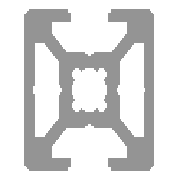
# Autodesk Inventor part: 3 842 993 422-25mm
Saved by Autodesk Inventor 2011 SP1 (Build 150282100, 282)
## iProperties
Created: 2011-02-10
Part Number: 3 842 993 422-25mm
Document SubType Name: Modeling
Designer: S. Wile
Density: 2.71 g/cm^3
Categories: <MemberInstance><Categories><Category DisplayName="Structural Shapes" InternalName="089c4875-fa83-4c05-b084-43b9cc11f5ed" Mnemonic="GRDR"><CategoryParameter DisplayName="Custom Base Point" InternalName="4f1d1b73-316d-484b-a3df-9cbabb16eb77" Mnemonic="shpBasePoint"/><CategoryParameter DisplayName="FG Authored" InternalName="9c666724-f362-4ea7-ac62-f6a007de5c69" Mnemonic="shpFGAuto"/><CategoryParameter DisplayName="Legacy Member ID" InternalName="340afe4f-75d7-48d3-ab7d-943f3c3da468" Mnemonic="LegacyMemberID"/><CategoryParameter DisplayName="Base Length" InternalName="42e34263-8f20-4d0e-ad48-bf1385b87c24" Mnemonic="shplen"/><CategoryParameter DisplayName="Distance of the Center of Gravity X-X" InternalName="26c9bdb8-9c79-4b4f-a92e-8e197583c9c4" Mnemonic="grcendistX"/><CategoryParameter DisplayName="Distance of the Center of Gravity Y-Y" InternalName="bcc4fb17-7af4-436a-8f8c-d0aa3b0248c5" Mnemonic="grcendistY"/><CategoryParameter DisplayName="Torsional Rigidity Modulus" InternalName="26c1ec35-5026-4c63-ad0a-751cf684a536" Mnemonic="torrigmod"/><CategoryParameter DisplayName="Torsional Section Modulus" InternalName="7c55a8dc-8844-49f9-a867-cc677b30ec9a" Mnemonic="torsecmod"/><CategoryParameter DisplayName="Coefficient of Shear Displacement" InternalName="de4c90c6-aaa8-468f-a335-6737b311b5d3" Mnemonic="shdispc"/><CategoryParameter DisplayName="Section Area" InternalName="1ff91680-64b0-4202-b9a3-7fd3f94bba3b" Mnemonic="secarea"/><CategoryParameter DisplayName="Moment of Inertia (x)" InternalName="4cd780bc-73d7-43ac-917a-579e5cbd684d" Mnemonic="inermomx"/><CategoryParameter DisplayName="Moment of Inertia (y)" InternalName="4b9f58ea-bced-460e-81ea-3d29ca5a49e3" Mnemonic="inermomy"/><CategoryParameter DisplayName="Section Module (x)" InternalName="72cfad18-cf51-4ed4-aaa7-c6b224f8419f" Mnemonic="secmodx"/><CategoryParameter DisplayName="Section Module (y)" InternalName="59eaa5e9-d227-48dc-b6c1-6920f96e0f95" Mnemonic="secmody"/><CategoryParameter DisplayName="Radius of Gyration (x)" InternalName="25778675-03e9-40c1-b6a8-4a9ed693320d" Mnemonic="gyrradx"/><CategoryParameter DisplayName="Radius of Gyration (y)" InternalName="bfa18ebe-1636-4dbe-8d42-b263e0b73184" Mnemonic="gyrrady"/><CategoryParameter DisplayName="Shape Thickness" InternalName="d109cf76-8eb4-42fc-9800-4409734adc67" Mnemonic="shpthick"/><CategoryParameter DisplayName="Second Shape Thickness" InternalName="9251a8e1-85fd-4e47-af99-afdb762317d9" Mnemonic="shpthick2"/><CategoryParameter DisplayName="Shape Width" InternalName="7c717d54-a18f-4666-b4d4-573cce22c62c" Mnemonic="shpwdth"/><CategoryParameter DisplayName="Shape Height" InternalName="50274e7d-5ac0-4796-92cb-c59e54983c67" Mnemonic="shpheig"/><CategoryParameter DisplayName="Mass per Length Unit" InternalName="0bb95a10-148f-4027-a459-38d7b056702a" Mnemonic="shpmass"/><CategoryParameter DisplayName="Section Designation" InternalName="5a64d034-428d-49c8-ba32-7619764de20f" Mnemonic="shpdes"/><Category DisplayName="Other" InternalName="f02205ff-2390-476f-921c-0b3185f88e84" Mnemonic="OTHSHP"><CategoryParameter DisplayName="Moment of Inertia (x)" InternalName="ec6737bc-264f-43ed-b0bd-f6d410c2718d" Mnemonic="inermomx"/><CategoryParameter DisplayName="Moment of Inertia (y)" InternalName="044c654e-f649-48ac-84cc-650a29ae31ca" Mnemonic="inermomy"/><CategoryParameter DisplayName="Section Module (x)" InternalName="cac70804-9d39-43bb-be17-56ea1f39a6c2" Mnemonic="secmodx"/><CategoryParameter DisplayName="Section Module (y)" InternalName="88b8bff9-a616-4028-93d5-ed4f79680d13" Mnemonic="secmody"/><CategoryParameter DisplayName="Section Area" InternalName="c46ecdf8-b6eb-4db9-8b25-30258930c1e3" Mnemonic="secarea"/><CategoryParameter DisplayName="Radius of Gyration (x)" InternalName="ee72c61e-565e-4fd6-b448-66e1e1abcb7e" Mnemonic="gyrradx"/><CategoryParameter DisplayName="Radius of Gyration (y)" InternalName="743e1dfe-1bba-408b-b985-cf752b207386" Mnemonic="gyrrady"/><CategoryParameter DisplayName="Shape Thickness" InternalName="12b1a788-9233-48fd-a933-2df8ff42b15f" Mnemonic="shpthick"/><CategoryParameter DisplayName="Mass per Length Unit" InternalName="2fd289d6-9394-4d2d-97e6-6659d7d4551d" Mnemonic="shpmass"/></Category></Category></Categories><FamilyTemplate Id="20x20-2S"><FamilyTemplateParameters><FamilyTemplateParameter ObjectType="kUserParameterObject" ValueType="xs:double" Id="1" ObjectReferenceKey="Length"/><FamilyTemplateParameter ObjectType="kPropertyObject" ValueType="xs:string" Id="4" ObjectReferenceKey="{32853F0F-3444-11d1-9E93-0060B03C1CA6}" SubObjectId="52"/><FamilyTemplateParameter ObjectType="kPartComponentDefinitionObject" ValueType="xs:string" Id="5" SubObjectId="Material"/><FamilyTemplateParameter ObjectType="kPropertyObject" ValueType="xs:string" Id="6" ObjectReferenceKey="{32853F0F-3444-11d1-9E93-0060B03C1CA6}" SubObjectId="5"/><FamilyTemplateParameter ObjectType="kPropertyObject" ValueType="xs:string" Id="7" ObjectReferenceKey="{32853F0F-3444-11D1-9E93-0060B03C1CA6}" SubObjectId="55"/><FamilyTemplateParameter ObjectType="kiPartTableColumnObject" ValueType="xs:string" Id="16" ObjectReferenceKey="FILENAME"/><FamilyTemplateParameter ObjectType="kiPartTableColumnObject" ValueType="xs:string" Id="17" ObjectReferenceKey="MEMBER_REVISION"/></FamilyTemplateParameters></FamilyTemplate><CategoryParameterMap><ParamToTemplateMap><ParamToTemplate CategoryParameter="//CategoryParameter[@InternalName='2675968c-4ce5-49e0-a4f5-552d29089031']" TemplateParameter="4"/><ParamToTemplate CategoryParameter="//CategoryParameter[@InternalName='8b46a4cc-9585-4fed-90c3-899f57e09a73']" TemplateParameter="16"/><ParamToTemplate CategoryParameter="//CategoryParameter[@InternalName='42e34263-8f20-4d0e-ad48-bf1385b87c24']" TemplateParameter="1"/><ParamToTemplate CategoryParameter="//CategoryParameter[@InternalName='818a152a-d3c3-49ca-80ee-df7d91421b8e']" TemplateParameter="5"/><ParamToTemplate CategoryParameter="//CategoryParameter[@InternalName='a65d44b9-392f-4f4f-857b-e4b3d54996fe']" TemplateParameter="17"/><ParamToTemplate CategoryParameter="//CategoryParameter[@InternalName='016b6077-bfbe-49bd-92c9-d8d59c39c941']" TemplateParameter="6"/><ParamToTemplate CategoryParameter="//CategoryParameter[@InternalName='9c666724-f362-4ea7-ac62-f6a007de5c69']" ConstantValue="1"/></ParamToTemplateMap></CategoryParameterMap></MemberInstance>
Stock Number: 3 842 993 422
Description: PROFILE 20x20 2S, -/-
Material: Aluminum-6061
Mass: 12.367 g
Surface Area: 53.0413 cm^2
Volume: 4.56348 cm^3
Author: S. Wile
Autodesk Inventor part; units mm, degrees
ref_plane "YZ Plane" through (0, 0, 0) normal (1, 0, 0) x (0, 1, 0)
ref_plane "XZ Plane" through (0, 0, 0) normal (0, 1, 0) x (-1, 0, 0)
ref_plane "XY Plane" through (0, 0, 0) normal (0, 0, 1) x (1, 0, 0)
sketch "20x20-2S" plane through (0, 0, 0) normal (0, 0, 1) x (1, 0, 0)
  line L0 (120.3777, 73.0122) -> (125.1777, 73.0122)
  line L1 (125.3777, 73.2122) -> (125.3777, 73.3122)
  line L2 (125.5777, 73.5122) -> (125.6777, 73.5122)
  line L3 (125.8777, 73.7122) -> (125.8777, 74.3122)
  line L4 (125.6777, 74.5122) -> (123.0777, 74.5122)
  line L5 (122.8777, 74.7122) -> (122.8777, 75.8794)
  line L6 (122.9363, 76.0208) -> (125.3691, 78.4537)
  line L7 (125.5105, 78.5122) -> (127.9045, 78.5122)
  line L8 (128.0045, 78.539) -> (128.7777, 78.9854)
  line L9 (128.9777, 78.9854) -> (129.7509, 78.539)
  line L10 (129.8509, 78.5122) -> (132.2449, 78.5122)
  line L11 (132.3863, 78.4537) -> (134.8191, 76.0208)
  line L12 (134.8777, 75.8794) -> (134.8777, 74.7122)
  line L13 (134.6777, 74.5122) -> (132.0777, 74.5122)
  line L14 (131.8777, 74.3122) -> (131.8777, 73.7122)
  line L15 (132.0777, 73.5122) -> (132.1777, 73.5122)
  line L16 (132.3777, 73.3122) -> (132.3777, 73.2122)
  line L17 (132.5777, 73.0122) -> (137.3777, 73.0122)
  arc A0 (137.3777, 73.0122) -> (138.8777, 74.5122) centre (137.3777, 74.5122) ccw
  line L18 (138.8777, 74.5122) -> (138.8777, 91.5122)
  arc A1 (138.8777, 91.5122) -> (137.3777, 93.0122) centre (137.3777, 91.5122) ccw
  arc A2 (126.9906, 85.9599) -> (125.9299, 84.8992) centre (128.8777, 83.0122) ccw
  line L19 (125.9299, 84.8992) -> (126.442, 84.2889)
  arc A3 (126.442, 84.2889) -> (126.442, 81.7355) centre (128.8777, 83.0122) ccw
  line L20 (126.442, 81.7355) -> (125.9299, 81.1252)
  arc A4 (125.9299, 81.1252) -> (126.9906, 80.0646) centre (128.8777, 83.0122) ccw
  line L21 (126.9906, 80.0646) -> (127.6009, 80.5766)
  arc A5 (127.6009, 80.5766) -> (130.1546, 80.5766) centre (128.8777, 83.0122) ccw
  line L22 (130.1546, 80.5766) -> (130.7648, 80.0646)
  arc A6 (130.7648, 80.0646) -> (131.8255, 81.1252) centre (128.8777, 83.0122) ccw
  line L23 (131.8255, 81.1252) -> (131.3134, 81.7355)
  arc A7 (131.3134, 81.7355) -> (131.3134, 84.2889) centre (128.8777, 83.0122) ccw
  line L24 (131.3134, 84.2889) -> (131.8255, 84.8992)
  arc A8 (131.8255, 84.8992) -> (130.7648, 85.9599) centre (128.8777, 83.0122) ccw
  line L25 (130.7648, 85.9599) -> (130.1546, 85.4478)
  arc A9 (130.1546, 85.4478) -> (127.6009, 85.4478) centre (128.8777, 83.0122) ccw
  line L26 (127.6009, 85.4478) -> (126.9906, 85.9599)
  line L27 (124.3777, 83.9318) -> (124.3777, 86.3687)
  line L28 (124.3191, 86.5102) -> (121.8756, 88.9537)
  line L29 (121.7342, 89.0122) -> (120.5777, 89.0122)
  line L30 (120.3777, 88.8122) -> (120.3777, 83.5854)
  line L31 (120.3509, 83.4854) -> (120.1354, 83.1122)
  line L32 (120.1354, 82.9122) -> (120.3509, 82.539)
  line L33 (120.3777, 82.439) -> (120.3777, 77.2122)
  line L34 (121.8756, 77.0708) -> (124.3191, 79.5143)
  line L35 (124.3777, 79.6557) -> (124.3777, 82.0926)
  line L36 (124.4045, 82.1926) -> (124.82, 82.9122)
  line L37 (124.82, 83.1122) -> (124.4045, 83.8318)
  line L38 (133.3777, 82.0926) -> (133.3777, 79.6557)
  line L39 (133.4363, 79.5143) -> (135.8798, 77.0708)
  line L40 (136.0212, 77.0122) -> (137.1777, 77.0122)
  line L41 (137.3777, 77.2122) -> (137.3777, 82.439)
  line L42 (137.4045, 82.539) -> (137.62, 82.9122)
  line L43 (137.62, 83.1122) -> (137.4045, 83.4854)
  line L44 (137.3777, 83.5854) -> (137.3777, 88.8122)
  line L45 (137.1777, 89.0122) -> (136.0212, 89.0122)
  line L46 (135.8798, 88.9537) -> (133.4363, 86.5102)
  line L47 (133.3777, 86.3687) -> (133.3777, 83.9318)
  line L48 (133.3509, 83.8318) -> (132.9354, 83.1122)
  line L49 (132.9354, 82.9122) -> (133.3509, 82.1926)
  line L50 (120.5777, 77.0122) -> (121.7342, 77.0122)
  line L51 (137.3777, 93.0122) -> (132.5777, 93.0122)
  line L52 (132.3777, 92.8122) -> (132.3777, 92.7122)
  line L53 (132.1777, 92.5122) -> (132.0777, 92.5122)
  line L54 (131.8777, 92.3122) -> (131.8777, 91.7122)
  line L55 (132.0777, 91.5122) -> (134.6777, 91.5122)
  line L56 (134.8777, 91.3122) -> (134.8777, 90.1451)
  line L57 (134.8191, 90.0037) -> (132.3863, 87.5708)
  line L58 (132.2449, 87.5122) -> (129.8509, 87.5122)
  line L59 (129.7509, 87.4854) -> (128.9777, 87.039)
  line L60 (128.7777, 87.039) -> (128.0045, 87.4854)
  line L61 (127.9045, 87.5122) -> (125.5105, 87.5122)
  line L62 (125.3691, 87.5708) -> (122.9363, 90.0037)
  line L63 (122.8777, 90.1451) -> (122.8777, 91.3122)
  line L64 (123.0777, 91.5122) -> (125.6777, 91.5122)
  line L65 (125.8777, 91.7122) -> (125.8777, 92.3122)
  line L66 (125.6777, 92.5122) -> (125.5777, 92.5122)
  line L67 (125.3777, 92.7122) -> (125.3777, 92.8122)
  line L68 (125.1777, 93.0122) -> (120.3777, 93.0122)
  arc A10 (120.3777, 93.0122) -> (118.8777, 91.5122) centre (120.3777, 91.5122) ccw
  line L69 (118.8777, 91.5122) -> (118.8777, 74.5122)
  arc A11 (118.8777, 74.5122) -> (120.3777, 73.0122) centre (120.3777, 74.5122) ccw
  arc A12 (125.3777, 92.8122) -> (125.1777, 93.0122) centre (125.1777, 92.8122) ccw
  arc A13 (125.3777, 92.7122) -> (125.5777, 92.5122) centre (125.5777, 92.7122) ccw
  arc A14 (125.8777, 92.3122) -> (125.6777, 92.5122) centre (125.6777, 92.3122) ccw
  arc A15 (125.6777, 91.5122) -> (125.8777, 91.7122) centre (125.6777, 91.7122) ccw
  arc A16 (123.0777, 91.5122) -> (122.8777, 91.3122) centre (123.0777, 91.3122) ccw
  arc A17 (122.8777, 90.1451) -> (122.9363, 90.0037) centre (123.0777, 90.1451) ccw
  arc A18 (120.5777, 89.0122) -> (120.3777, 88.8122) centre (120.5777, 88.8122) ccw
  arc A19 (121.8756, 88.9537) -> (121.7342, 89.0122) centre (121.7342, 88.8122) ccw
  arc A20 (125.3691, 87.5708) -> (125.5105, 87.5122) centre (125.5105, 87.7122) ccw
  arc A21 (124.3777, 86.3687) -> (124.3191, 86.5102) centre (124.1777, 86.3687) ccw
  arc A22 (124.82, 82.9122) -> (124.82, 83.1122) centre (124.6468, 83.0122) ccw
  arc A23 (124.3777, 83.9318) -> (124.4045, 83.8318) centre (124.5777, 83.9318) ccw
  arc A24 (120.3509, 83.4854) -> (120.3777, 83.5854) centre (120.1777, 83.5854) ccw
  arc A25 (120.1354, 83.1122) -> (120.1354, 82.9122) centre (120.3086, 83.0122) ccw
  arc A26 (120.3777, 82.439) -> (120.3509, 82.539) centre (120.1777, 82.439) ccw
  arc A27 (124.4045, 82.1926) -> (124.3777, 82.0926) centre (124.5777, 82.0926) ccw
  arc A28 (128.7777, 87.039) -> (128.9777, 87.039) centre (128.8777, 87.2122) ccw
  arc A29 (128.0045, 87.4854) -> (127.9045, 87.5122) centre (127.9045, 87.3122) ccw
  arc A30 (129.8509, 87.5122) -> (129.7509, 87.4854) centre (129.8509, 87.3122) ccw
  arc A31 (132.2449, 87.5122) -> (132.3863, 87.5708) centre (132.2449, 87.7122) ccw
  arc A32 (134.8191, 90.0037) -> (134.8777, 90.1451) centre (134.6777, 90.1451) ccw
  arc A33 (134.8777, 91.3122) -> (134.6777, 91.5122) centre (134.6777, 91.3122) ccw
  arc A34 (131.8777, 91.7122) -> (132.0777, 91.5122) centre (132.0777, 91.7122) ccw
  arc A35 (132.0777, 92.5122) -> (131.8777, 92.3122) centre (132.0777, 92.3122) ccw
  arc A36 (132.1777, 92.5122) -> (132.3777, 92.7122) centre (132.1777, 92.7122) ccw
  arc A37 (132.5777, 93.0122) -> (132.3777, 92.8122) centre (132.5777, 92.8122) ccw
  arc A38 (136.0212, 89.0122) -> (135.8798, 88.9537) centre (136.0212, 88.8122) ccw
  arc A39 (137.3777, 88.8122) -> (137.1777, 89.0122) centre (137.1777, 88.8122) ccw
  arc A40 (133.4363, 86.5102) -> (133.3777, 86.3687) centre (133.5777, 86.3687) ccw
  arc A41 (133.3509, 83.8318) -> (133.3777, 83.9318) centre (133.1777, 83.9318) ccw
  arc A42 (132.9354, 83.1122) -> (132.9354, 82.9122) centre (133.1086, 83.0122) ccw
  arc A43 (133.3777, 82.0926) -> (133.3509, 82.1926) centre (133.1777, 82.0926) ccw
  arc A44 (137.4045, 82.539) -> (137.3777, 82.439) centre (137.5777, 82.439) ccw
  arc A45 (137.62, 82.9122) -> (137.62, 83.1122) centre (137.4468, 83.0122) ccw
  arc A46 (137.3777, 83.5854) -> (137.4045, 83.4854) centre (137.5777, 83.5854) ccw
  arc A47 (133.3777, 79.6557) -> (133.4363, 79.5143) centre (133.5777, 79.6557) ccw
  arc A48 (132.3863, 78.4537) -> (132.2449, 78.5122) centre (132.2449, 78.3122) ccw
  arc A49 (129.7509, 78.539) -> (129.8509, 78.5122) centre (129.8509, 78.7122) ccw
  arc A50 (137.1777, 77.0122) -> (137.3777, 77.2122) centre (137.1777, 77.2122) ccw
  arc A51 (135.8798, 77.0708) -> (136.0212, 77.0122) centre (136.0212, 77.2122) ccw
  arc A52 (134.8777, 75.8794) -> (134.8191, 76.0208) centre (134.6777, 75.8794) ccw
  arc A53 (134.6777, 74.5122) -> (134.8777, 74.7122) centre (134.6777, 74.7122) ccw
  arc A54 (132.0777, 74.5122) -> (131.8777, 74.3122) centre (132.0777, 74.3122) ccw
  arc A55 (131.8777, 73.7122) -> (132.0777, 73.5122) centre (132.0777, 73.7122) ccw
  arc A56 (132.3777, 73.3122) -> (132.1777, 73.5122) centre (132.1777, 73.3122) ccw
  arc A57 (132.3777, 73.2122) -> (132.5777, 73.0122) centre (132.5777, 73.2122) ccw
  arc A58 (125.1777, 73.0122) -> (125.3777, 73.2122) centre (125.1777, 73.2122) ccw
  arc A59 (125.5777, 73.5122) -> (125.3777, 73.3122) centre (125.5777, 73.3122) ccw
  arc A60 (125.6777, 73.5122) -> (125.8777, 73.7122) centre (125.6777, 73.7122) ccw
  arc A61 (125.8777, 74.3122) -> (125.6777, 74.5122) centre (125.6777, 74.3122) ccw
  arc A62 (127.9045, 78.5122) -> (128.0045, 78.539) centre (127.9045, 78.7122) ccw
  arc A63 (128.9777, 78.9854) -> (128.7777, 78.9854) centre (128.8777, 78.8122) ccw
  arc A64 (122.8777, 74.7122) -> (123.0777, 74.5122) centre (123.0777, 74.7122) ccw
  arc A65 (122.9363, 76.0208) -> (122.8777, 75.8794) centre (123.0777, 75.8794) ccw
  arc A66 (125.5105, 78.5122) -> (125.3691, 78.4537) centre (125.5105, 78.3122) ccw
  arc A67 (124.3191, 79.5143) -> (124.3777, 79.6557) centre (124.1777, 79.6557) ccw
  arc A68 (121.7342, 77.0122) -> (121.8756, 77.0708) centre (121.7342, 77.2122) ccw
  arc A69 (120.3777, 77.2122) -> (120.5777, 77.0122) centre (120.5777, 77.2122) ccw
  dimension "d0" = 0.2
  dimension "d1" = 0.2
  measures "d0" radius of A12
  measures "d1" radius of A58
sketch "Sketch1" plane through (0, 0, 0) normal (0, 0, 1) x (1, 0, 0)
  line L0 (-8.5, -10) -> (-3.7, -10)
  line L1 (-3.5, -9.8) -> (-3.5, -9.7)
  line L2 (-3.3, -9.5) -> (-3.2, -9.5)
  line L3 (-3, -9.3) -> (-3, -8.7)
  line L4 (-3.2, -8.5) -> (-5.8, -8.5)
  line L5 (-6, -8.3) -> (-6, -7.1328)
  line L6 (-5.9414, -6.9914) -> (-3.5086, -4.5586)
  line L7 (-3.3672, -4.5) -> (-0.9732, -4.5)
  line L8 (-0.8732, -4.4732) -> (-0.1, -4.0268)
  line L9 (0.1, -4.0268) -> (0.8732, -4.4732)
  line L10 (0.9732, -4.5) -> (3.3672, -4.5)
  line L11 (3.5086, -4.5586) -> (5.9414, -6.9914)
  line L12 (6, -7.1328) -> (6, -8.3)
  line L13 (5.8, -8.5) -> (3.2, -8.5)
  line L14 (3, -8.7) -> (3, -9.3)
  line L15 (3.2, -9.5) -> (3.3, -9.5)
  line L16 (3.5, -9.7) -> (3.5, -9.8)
  line L17 (3.7, -10) -> (8.5, -10)
  arc A0 (8.5, -10) -> (10, -8.5) centre (8.5, -8.5) ccw
  line L18 (10, -8.5) -> (10, 8.5)
  arc A1 (10, 8.5) -> (8.5, 10) centre (8.5, 8.5) ccw
  arc A2 (-1.8871, 2.9477) -> (-2.9478, 1.887) centre (0, 0) ccw
  line L19 (-2.9478, 1.887) -> (-2.4357, 1.2767)
  arc A3 (-2.4357, 1.2767) -> (-2.4357, -1.2767) centre (0, 0) ccw
  line L20 (-2.4357, -1.2767) -> (-2.9478, -1.887)
  arc A4 (-2.9478, -1.887) -> (-1.8871, -2.9477) centre (0, 0) ccw
  line L21 (-1.8871, -2.9477) -> (-1.2769, -2.4356)
  arc A5 (-1.2769, -2.4356) -> (1.2769, -2.4356) centre (0, 0) ccw
  line L22 (1.2769, -2.4356) -> (1.8871, -2.9477)
  arc A6 (1.8871, -2.9477) -> (2.9478, -1.887) centre (0, 0) ccw
  line L23 (2.9478, -1.887) -> (2.4357, -1.2767)
  arc A7 (2.4357, -1.2767) -> (2.4357, 1.2767) centre (0, 0) ccw
  line L24 (2.4357, 1.2767) -> (2.9478, 1.887)
  arc A8 (2.9478, 1.887) -> (1.8871, 2.9477) centre (0, 0) ccw
  line L25 (1.8871, 2.9477) -> (1.2769, 2.4356)
  arc A9 (1.2769, 2.4356) -> (-1.2769, 2.4356) centre (0, 0) ccw
  line L26 (-1.2769, 2.4356) -> (-1.8871, 2.9477)
  line L27 (-4.5, 0.9196) -> (-4.5, 3.3565)
  line L28 (-4.5586, 3.4979) -> (-7.0021, 5.9414)
  line L29 (-7.1435, 6) -> (-8.3, 6)
  line L30 (-8.5, 5.8) -> (-8.5, 0.5732)
  line L31 (-8.5268, 0.4732) -> (-8.7423, 0.1)
  line L32 (-8.7423, -0.1) -> (-8.5268, -0.4732)
  line L33 (-8.5, -0.5732) -> (-8.5, -5.8)
  line L34 (-7.0021, -5.9414) -> (-4.5586, -3.4979)
  line L35 (-4.5, -3.3565) -> (-4.5, -0.9196)
  line L36 (-4.4732, -0.8196) -> (-4.0577, -0.1)
  line L37 (-4.0577, 0.1) -> (-4.4732, 0.8196)
  line L38 (4.5, -0.9196) -> (4.5, -3.3565)
  line L39 (4.5586, -3.4979) -> (7.0021, -5.9414)
  line L40 (7.1435, -6) -> (8.3, -6)
  line L41 (8.5, -5.8) -> (8.5, -0.5732)
  line L42 (8.5268, -0.4732) -> (8.7423, -0.1)
  line L43 (8.7423, 0.1) -> (8.5268, 0.4732)
  line L44 (8.5, 0.5732) -> (8.5, 5.8)
  line L45 (8.3, 6) -> (7.1435, 6)
  line L46 (7.0021, 5.9414) -> (4.5586, 3.4979)
  line L47 (4.5, 3.3565) -> (4.5, 0.9196)
  line L48 (4.4732, 0.8196) -> (4.0577, 0.1)
  line L49 (4.0577, -0.1) -> (4.4732, -0.8196)
  line L50 (-8.3, -6) -> (-7.1435, -6)
  line L51 (8.5, 10) -> (3.7, 10)
  line L52 (3.5, 9.8) -> (3.5, 9.7)
  line L53 (3.3, 9.5) -> (3.2, 9.5)
  line L54 (3, 9.3) -> (3, 8.7)
  line L55 (3.2, 8.5) -> (5.8, 8.5)
  line L56 (6, 8.3) -> (6, 7.1328)
  line L57 (5.9414, 6.9914) -> (3.5086, 4.5586)
  line L58 (3.3672, 4.5) -> (0.9732, 4.5)
  line L59 (0.8732, 4.4732) -> (0.1, 4.0268)
  line L60 (-0.1, 4.0268) -> (-0.8732, 4.4732)
  line L61 (-0.9732, 4.5) -> (-3.3672, 4.5)
  line L62 (-3.5086, 4.5586) -> (-5.9414, 6.9914)
  line L63 (-6, 7.1328) -> (-6, 8.3)
  line L64 (-5.8, 8.5) -> (-3.2, 8.5)
  line L65 (-3, 8.7) -> (-3, 9.3)
  line L66 (-3.2, 9.5) -> (-3.3, 9.5)
  line L67 (-3.5, 9.7) -> (-3.5, 9.8)
  line L68 (-3.7, 10) -> (-8.5, 10)
  arc A10 (-8.5, 10) -> (-10, 8.5) centre (-8.5, 8.5) ccw
  line L69 (-10, 8.5) -> (-10, -8.5)
  arc A11 (-10, -8.5) -> (-8.5, -10) centre (-8.5, -8.5) ccw
  arc A12 (-3.5, 9.8) -> (-3.7, 10) centre (-3.7, 9.8) ccw
  arc A13 (-3.5, 9.7) -> (-3.3, 9.5) centre (-3.3, 9.7) ccw
  arc A14 (-3, 9.3) -> (-3.2, 9.5) centre (-3.2, 9.3) ccw
  arc A15 (-3.2, 8.5) -> (-3, 8.7) centre (-3.2, 8.7) ccw
  arc A16 (-5.8, 8.5) -> (-6, 8.3) centre (-5.8, 8.3) ccw
  arc A17 (-6, 7.1328) -> (-5.9414, 6.9914) centre (-5.8, 7.1328) ccw
  arc A18 (-8.3, 6) -> (-8.5, 5.8) centre (-8.3, 5.8) ccw
  arc A19 (-7.0021, 5.9414) -> (-7.1435, 6) centre (-7.1435, 5.8) ccw
  arc A20 (-3.5086, 4.5586) -> (-3.3672, 4.5) centre (-3.3672, 4.7) ccw
  arc A21 (-4.5, 3.3565) -> (-4.5586, 3.4979) centre (-4.7, 3.3565) ccw
  arc A22 (-4.0577, -0.1) -> (-4.0577, 0.1) centre (-4.2309, 0) ccw
  arc A23 (-4.5, 0.9196) -> (-4.4732, 0.8196) centre (-4.3, 0.9196) ccw
  arc A24 (-8.5268, 0.4732) -> (-8.5, 0.5732) centre (-8.7, 0.5732) ccw
  arc A25 (-8.7423, 0.1) -> (-8.7423, -0.1) centre (-8.5691, 0) ccw
  arc A26 (-8.5, -0.5732) -> (-8.5268, -0.4732) centre (-8.7, -0.5732) ccw
  arc A27 (-4.4732, -0.8196) -> (-4.5, -0.9196) centre (-4.3, -0.9196) ccw
  arc A28 (-0.1, 4.0268) -> (0.1, 4.0268) centre (0, 4.2) ccw
  arc A29 (-0.8732, 4.4732) -> (-0.9732, 4.5) centre (-0.9732, 4.3) ccw
  arc A30 (0.9732, 4.5) -> (0.8732, 4.4732) centre (0.9732, 4.3) ccw
  arc A31 (3.3672, 4.5) -> (3.5086, 4.5586) centre (3.3672, 4.7) ccw
  arc A32 (5.9414, 6.9914) -> (6, 7.1328) centre (5.8, 7.1328) ccw
  arc A33 (6, 8.3) -> (5.8, 8.5) centre (5.8, 8.3) ccw
  arc A34 (3, 8.7) -> (3.2, 8.5) centre (3.2, 8.7) ccw
  arc A35 (3.2, 9.5) -> (3, 9.3) centre (3.2, 9.3) ccw
  arc A36 (3.3, 9.5) -> (3.5, 9.7) centre (3.3, 9.7) ccw
  arc A37 (3.7, 10) -> (3.5, 9.8) centre (3.7, 9.8) ccw
  arc A38 (7.1435, 6) -> (7.0021, 5.9414) centre (7.1435, 5.8) ccw
  arc A39 (8.5, 5.8) -> (8.3, 6) centre (8.3, 5.8) ccw
  arc A40 (4.5586, 3.4979) -> (4.5, 3.3565) centre (4.7, 3.3565) ccw
  arc A41 (4.4732, 0.8196) -> (4.5, 0.9196) centre (4.3, 0.9196) ccw
  arc A42 (4.0577, 0.1) -> (4.0577, -0.1) centre (4.2309, 0) ccw
  arc A43 (4.5, -0.9196) -> (4.4732, -0.8196) centre (4.3, -0.9196) ccw
  arc A44 (8.5268, -0.4732) -> (8.5, -0.5732) centre (8.7, -0.5732) ccw
  arc A45 (8.7423, -0.1) -> (8.7423, 0.1) centre (8.5691, 0) ccw
  arc A46 (8.5, 0.5732) -> (8.5268, 0.4732) centre (8.7, 0.5732) ccw
  arc A47 (4.5, -3.3565) -> (4.5586, -3.4979) centre (4.7, -3.3565) ccw
  arc A48 (3.5086, -4.5586) -> (3.3672, -4.5) centre (3.3672, -4.7) ccw
  arc A49 (0.8732, -4.4732) -> (0.9732, -4.5) centre (0.9732, -4.3) ccw
  arc A50 (8.3, -6) -> (8.5, -5.8) centre (8.3, -5.8) ccw
  arc A51 (7.0021, -5.9414) -> (7.1435, -6) centre (7.1435, -5.8) ccw
  arc A52 (6, -7.1328) -> (5.9414, -6.9914) centre (5.8, -7.1328) ccw
  arc A53 (5.8, -8.5) -> (6, -8.3) centre (5.8, -8.3) ccw
  arc A54 (3.2, -8.5) -> (3, -8.7) centre (3.2, -8.7) ccw
  arc A55 (3, -9.3) -> (3.2, -9.5) centre (3.2, -9.3) ccw
  arc A56 (3.5, -9.7) -> (3.3, -9.5) centre (3.3, -9.7) ccw
  arc A57 (3.5, -9.8) -> (3.7, -10) centre (3.7, -9.8) ccw
  arc A58 (-3.7, -10) -> (-3.5, -9.8) centre (-3.7, -9.8) ccw
  arc A59 (-3.3, -9.5) -> (-3.5, -9.7) centre (-3.3, -9.7) ccw
  arc A60 (-3.2, -9.5) -> (-3, -9.3) centre (-3.2, -9.3) ccw
  arc A61 (-3, -8.7) -> (-3.2, -8.5) centre (-3.2, -8.7) ccw
  arc A62 (-0.9732, -4.5) -> (-0.8732, -4.4732) centre (-0.9732, -4.3) ccw
  arc A63 (0.1, -4.0268) -> (-0.1, -4.0268) centre (0, -4.2) ccw
  arc A64 (-6, -8.3) -> (-5.8, -8.5) centre (-5.8, -8.3) ccw
  arc A65 (-5.9414, -6.9914) -> (-6, -7.1328) centre (-5.8, -7.1328) ccw
  arc A66 (-3.3672, -4.5) -> (-3.5086, -4.5586) centre (-3.3672, -4.7) ccw
  arc A67 (-4.5586, -3.4979) -> (-4.5, -3.3565) centre (-4.7, -3.3565) ccw
  arc A68 (-7.1435, -6) -> (-7.0021, -5.9414) centre (-7.1435, -5.8) ccw
  arc A69 (-8.5, -5.8) -> (-8.3, -6) centre (-8.3, -5.8) ccw
  constraints: 1 other
extrude "Extrusion3" add sketch "Sketch1" along normal blind 30
body "Solid2"
